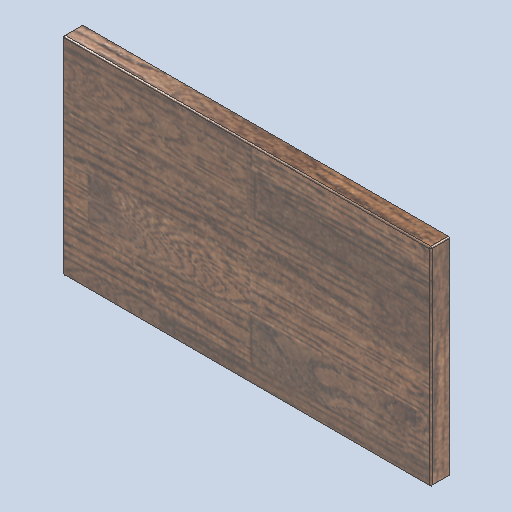
# Autodesk Inventor part: Drawer Front Panel
Saved by Autodesk Inventor 2022 (Build 260153000, 153)
## iProperties
Company: Jay's Dressers
RuleStatus: InUse
Created: 2021-10-04
Material: Generic
Document SubType Name: Modeling
Designer: Admin
Density: 1 g/cm^3
Appearance: White Ash - Java
Author: Admin
Title: Drawer Front Panel
Autodesk Inventor part; units mm, degrees
ref_plane "YZ Plane" through (0, 0, 0) normal (1, 0, 0) x (0, 1, 0)
ref_plane "XZ Plane" through (0, 0, 0) normal (0, 1, 0) x (-1, 0, 0)
ref_plane "XY Plane" through (0, 0, 0) normal (0, 0, 1) x (1, 0, 0)
derived "Dresser SKELETON.ipt"
sketch "Sketch1" plane through (0, 0, 0) normal (0, 0, 1) x (1, 0, 0)
  line L0 (247.65, -139.7) -> (-247.65, -139.7)
  line L1 (-247.65, -139.7) -> (-247.65, 139.7)
  line L2 (-247.65, 139.7) -> (247.65, 139.7)
  line L3 (247.65, 139.7) -> (247.65, -139.7)
  line L4 (247.65, -139.7) -> (-247.65, 139.7) construction
  line L5 (-247.65, -139.7) -> (247.65, 139.7) construction
  point P0 (0, 0)
  dimension "d1" = 495.3
  dimension "d2" = 279.4
  constraints: 12 end point, 2 midpoint, 2 parallel, 1 horizontal, 1 perpendicular
  measures "d1" distance of L1.end L2.end
  measures "d2" distance of L0.end L1.end
extrude "Extrusion1" add sketch "Sketch1" along normal blind 25.4
fillet "Fillet1" radius 1.905 8 edges at (-247.65, 0, 25.4) (0, -139.7, 25.4) (0, 139.7, 25.4) (247.65, 0, 25.4) (247.65, 139.7, 12.7) (-247.65, 139.7, 12.7) (247.65, -139.7, 12.7) (-247.65, -139.7, 12.7)
sketch "Sketch2" plane through (0, 0, 0) normal (1, 0, 0) x (0, 1, 0)
  line L0 (139.7, 0) -> (139.7, 25.4)
  line L1 (139.7, 25.4) -> (120.65, 25.4)
  arc A0 (120.65, 25.4) -> (139.7, 6.35) centre (139.7, 25.4) ccw
  point P0 (0, 0)
  point P1 (139.7, 0)
  point P2 (139.7, 0)
  point P3 (139.7, 0)
  dimension "d7" = 25.4
  dimension "d8" = 19.05
  constraints: 4 end point, 2 point on circle, 2 point on line, 1 centre point, 1 coincident, 1 horizontal, 1 line through centre, 1 vertical
  measures "d7" distance of L0.start L0.end
  measures "d8" distance of L0.end L1.end
feature "Elegant Sweep" [suppressed]
fillet "Elegant Fillet" [suppressed]
chamfer "Elegant Chamfer" [suppressed]
equation "\"d3\" = panelThickness"
equation "\"d7\" = panelThickness"
equation "\"panelThickness\" = 25.4"
body "Solid1"
